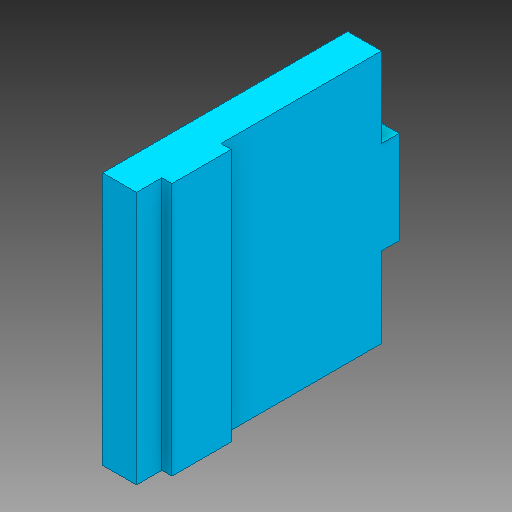
# Autodesk Inventor part: gamma
Saved by Autodesk Inventor 2018 (Build 220112000, 112)
## iProperties
Created: 2018-06-03
Part Number: gamma
Material: Všeobecné
Document SubType Name: Modeling
Designer: Kuba
Density: 1 g/cm^3
Appearance: Výchozí
Mass: 3.8244 g
Surface Area: 23.638 cm^2
Volume: 3.8244 cm^3
Author: Kuba
Autodesk Inventor part; units mm, degrees
ref_plane "YZ Plane" through (0, 0, 0) normal (1, 0, 0) x (0, 1, 0)
ref_plane "XZ Plane" through (0, 0, 0) normal (0, 1, 0) x (-1, 0, 0)
ref_plane "XY Plane" through (0, 0, 0) normal (0, 0, 1) x (1, 0, 0)
sketch "Náčrt1" plane through (0, 0, 0) normal (1, 0, 0) x (0, 1, 0)
  line L0 (14.5, 15) -> (-14.5, 15)
  line L1 (-14.5, 15) -> (-14.5, -15)
  line L2 (-14.5, -15) -> (14.5, -15)
  line L3 (14.5, -15) -> (14.5, 15)
  line L4 (14.5, 5.5) -> (16.6, 5.5)
  line L5 (16.6, 5.5) -> (16.6, -5.5)
  line L6 (16.6, -5.5) -> (14.5, -5.5)
  line L7 (14.5, -5.5) -> (14.5, 5.5)
  point P0 (0, 0)
  dimension "d0" = 29
  dimension "d1" = 30
  dimension "d2" = 2.1
  dimension "d3" = 11
  dimension "d4" = 15
  dimension "d5" = 14.5
  dimension "d6" = 5.5
  constraints: 16 end point, 4 parallel, 2 horizontal, 2 perpendicular, 1 point on line
  measures "d0" distance of L0.start L0.end
  measures "d1" distance of L2.end L0.start
  measures "d2" distance of L4.start L4.end
  measures "d3" distance of L4.end L5.end
  measures "d4" distance from line of L0 point (0, 0)
  measures "d5" distance from line of L1 point (0, 0)
  measures "d6" distance from line of point (0, 0) L6
extrude "Vysunutí1" add sketch "Náčrt1" along normal blind 4
sketch "Náčrt2" plane through (4, 0, 0) normal (1, 0, 0) x (0, 0, -1)
  line L0 (-15, -4.5) -> (15, -4.5)
  line L1 (15, -4.5) -> (15, -11.5)
  line L2 (15, -11.5) -> (-15, -11.5)
  line L3 (-15, -11.5) -> (-15, -4.5)
  line L4 (5.5, 14.5) -> (5.5, 16.6) projected
  line L5 (5.5, 16.6) -> (-5.5, 16.6) projected
  line L6 (-5.5, 16.6) -> (-5.5, 14.5) projected
  line L7 (-5.5, 14.5) -> (-15, 14.5) projected
  line L8 (-15, 14.5) -> (-15, -14.5) projected
  line L9 (-15, -14.5) -> (15, -14.5) projected
  line L10 (15, -14.5) -> (15, 14.5) projected
  line L11 (15, 14.5) -> (5.5, 14.5) projected
  line L12 (-15, 14.5) -> (-15, -14.5) projected
  line L13 (15, -14.5) -> (15, 14.5) projected
  point P0 (0, 0)
  dimension "d9" = 10
  dimension "d10" = 3
  constraints: 8 end point, 2 collinear, 2 parallel, 1 horizontal, 1 perpendicular
  measures "d9" distance between parallel lines of L9 L0
  measures "d10" distance between parallel lines of L9 L2
extrude "Vysunutí2" add sketch "Náčrt2" along normal blind 1.2 contours L0 L1 L2 L3
equation "\"d4\" = 0.5 * d1"
equation "\"d5\" = 0.5 * d0"
equation "\"d6\" = 0.5 * d3"
